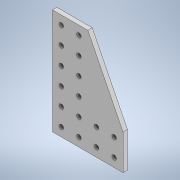
# Autodesk Inventor part: 6x4
Saved by Autodesk Inventor 2020 (Build 240168000, 168)
## iProperties
Created: 2020-01-13
Part Number: 6x4
Material: Generic
Document SubType Name: Modeling
Designer: 339294
Density: 1 g/cm^3
Appearance: Default
Author: 339294
Autodesk Inventor part; units mm, degrees
ref_plane "YZ Plane" through (0, 0, 0) normal (1, 0, 0) x (0, 1, 0)
ref_plane "XZ Plane" through (0, 0, 0) normal (0, 1, 0) x (-1, 0, 0)
ref_plane "XY Plane" through (0, 0, 0) normal (0, 0, 1) x (1, 0, 0)
sketch "Sketch1" plane through (0, 0, 0) normal (0, 0, 1) x (1, 0, 0)
  line L0 (0, 0) -> (101.6, 0)
  line L1 (101.6, 0) -> (101.6, 50.8)
  line L2 (0, 50.8) -> (0, 0)
  line L3 (50.8, 152.4) -> (0, 152.4)
  line L4 (0, 152.4) -> (0, 50.8)
  line L5 (50.8, 152.4) -> (101.6, 50.8)
  circle A0 centre (12.7, 12.7) radius 3.2512
  circle A1 centre (12.7, 38.1) radius 3.2512
  circle A2 centre (12.7, 63.5) radius 3.2512
  circle A3 centre (12.7, 88.9) radius 3.2512
  circle A4 centre (12.7, 114.3) radius 3.2512
  circle A5 centre (12.7, 139.7) radius 3.2512
  circle A6 centre (38.1, 12.7) radius 3.2512
  circle A7 centre (38.1, 38.1) radius 3.2512
  circle A8 centre (38.1, 63.5) radius 3.2512
  circle A9 centre (38.1, 88.9) radius 3.2512
  circle A10 centre (38.1, 114.3) radius 3.2512
  circle A11 centre (38.1, 139.7) radius 3.2512
  circle A12 centre (63.5, 12.7) radius 3.2512
  circle A13 centre (88.9, 12.7) radius 3.2512
  circle A14 centre (38.1, 38.1) radius 3.2512
  circle A15 centre (63.5, 38.1) radius 3.2512
  circle A16 centre (88.9, 38.1) radius 3.2512
  dimension "d6" = 101.6
  dimension "d7" = 50.8
  dimension "d8" = 50.8
  dimension "d9" = 101.6
  dimension "d10" = 50.8
  dimension "d11" = 101.6
  dimension "d12" = 50.8
  dimension "d13" = 6.5024
  dimension "d14" = 12.7
  dimension "d15" = 12.7
  dimension "d18" = 25.4
  dimension "d21" = 25.4
  dimension "d26" = 25.4
  dimension "d29" = 25.4
  constraints: 17 centre point, 12 end point, 3 horizontal, 2 vertical, 1 parallel, 1 perpendicular, 32 other
  measures "d6" distance of L3.end L2.start
  measures "d7" distance of L2.start L0.start
  measures "d8" distance of L3.start L3.end
  measures "d9" vertical distance of L3.start L1.end
  measures "d10" distance of L0.end L1.end
  measures "d11" distance of L0.start L0.end
  measures "d12" horizontal distance of L3.start L1.end
  measures "d13" diameter of A0
  measures "d14" distance from line of L0 A0.centre
  measures "d15" distance from line of L2 A0.centre
  measures "d18" distance of A0.centre A1.centre
  measures "d21" distance of A0.centre A6.centre
  measures "d26" distance of A6.centre A12.centre
  measures "d29" distance of A6.centre A14.centre
extrude "Extrusion1" add sketch "Sketch1" along normal blind 6.35
body "Solid1"
